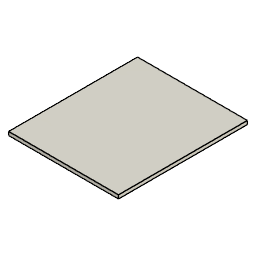
Produs Final 3D (Autodesk Fusion 360 archive; units mm, degrees)
design "Display_3D"
part number: 2026-04-13-22-43-48-717
Autodesk Fusion 360 part; units mm, degrees
sketch "Sketch1" plane through (0, 0, 0) normal (0, 0, 1) x (1, 0, 0)
  line L0 (-25, 25) -> (6.8, 25)
  line L1 (6.8, 25) -> (6.8, -12.32)
  line L2 (6.8, -12.32) -> (-25, -12.32)
  line L3 (-25, -12.32) -> (-25, 25)
  dimension "d1" = 31.8
  dimension "d2" = 37.32
  constraint horizontal L0
  constraint vertical L1
  constraint horizontal L2
  constraint vertical L3
  measures "d1" distance of L0.start L0.end
  measures "d2" distance of L0.start L2.end
extrude "Extrude1" add sketch "Sketch1" along normal blind 1.05

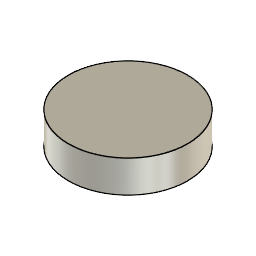
design "Shaker_3D"
part number: 2026-04-13-22-51-33-639
Autodesk Fusion 360 part; units mm, degrees
sketch "Sketch1" plane through (0, 0, 0) normal (0, 0, 1) x (1, 0, 0)
  circle A0 centre (-41.6124, 34.0465) radius 5
  dimension "d1" = 10
  measures "d1" diameter of A0
extrude "Extrude1" add sketch "Sketch1" along normal blind 2.7

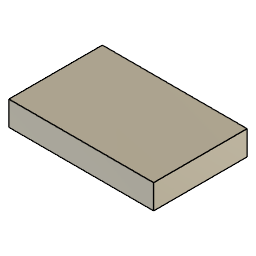
design "Baterie_3D"
part number: 2026-04-13-22-34-44-768
Autodesk Fusion 360 part; units mm, degrees
sketch "Sketch1" plane through (0, 0, 0) normal (0, 0, 1) x (1, 0, 0)
  line L0 (-50, 50) -> (-17.5, 50)
  line L1 (-17.5, 50) -> (-17.5, 29)
  line L2 (-17.5, 29) -> (-50, 29)
  line L3 (-50, 29) -> (-50, 50)
  dimension "d1" = 32.5
  dimension "d2" = 21
  constraint horizontal L0
  constraint vertical L1
  constraint horizontal L2
  constraint vertical L3
  measures "d1" distance of L0.start L0.end
  measures "d2" distance of L0.start L2.end
extrude "Extrude1" add sketch "Sketch1" along normal blind 5.5
